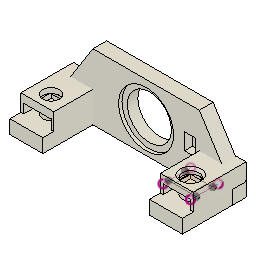
encoder-bracket (Autodesk Fusion 360 design; units mm, degrees)
Autodesk Fusion 360 part; units mm, degrees
sketch "Sketch1" plane through (0, 0, 0) normal (0, 0, 1) x (1, 0, 0)
  line L0 (-19.939, 0) -> (-19.939, 3.175)
  line L1 (-19.939, 3.175) -> (-12.319, 15.24)
  line L2 (-12.319, 15.24) -> (12.319, 15.24)
  line L3 (12.319, 15.24) -> (19.939, 3.175)
  line L4 (19.939, 3.175) -> (19.939, 0)
  line L5 (19.939, 0) -> (-19.939, 0)
  line L6 (0, 0) -> (0, 15.24) construction
  circle A0 centre (0, 7.3025) radius 5.08
  circle A1 centre (0, 7.3025) radius 6.35
  line L7 (8.89, 9.2075) -> (11.43, 9.2075)
  line L8 (11.43, 9.2075) -> (11.43, 5.3975)
  line L9 (11.43, 5.3975) -> (8.89, 5.3975)
  line L10 (8.89, 5.3975) -> (8.89, 9.2075)
  line L11 (10.16, 9.2075) -> (10.16, 5.3975) construction
  line L12 (0, 7.3025) -> (10.16, 7.3025) construction
  dimension "d1" = 39.878
  dimension "d2" = 3.175
  dimension "d3" = 7.62
  dimension "d4" = 15.24
  dimension "d5" = 10.16
  dimension "d6" = 7.3025
  dimension "d7" = 12.7
  dimension "d8" = 3.81
  dimension "d9" = 2.54
  dimension "d10" = 10.16
  constraint vertical L0
  constraint perpendicular L0 L2
  constraint perpendicular L2 L4
  constraint perpendicular L0 L5
  constraint midpoint L6.start L5
  constraint equal L0 L4
  constraint coincident L6.start origin
  constraint coincident L2 L6.end
  constraint perpendicular L2 L6
  constraint midpoint L2 L6.end
  constraint coincident L6 A0.centre
  constraint concentric A0 A1
  constraint horizontal L7
  constraint vertical L8
  constraint horizontal L9
  constraint vertical L10
  constraint midpoint L7 L11.start
  constraint midpoint L9 L11.end
  constraint coincident A0.centre A1.centre
  constraint coincident L11 L12.end
  constraint perpendicular L11 L12
  constraint midpoint L11 L12.end
  measures "d1" distance of L0.start L4.end
  measures "d2" distance of L0.start L0.end
  measures "d3" horizontal distance of L0.start L1.end
  measures "d4" distance of L2 L5
  measures "d5" diameter of A0
  measures "d6" distance of L6.start A0.centre
  measures "d7" diameter of A1
  measures "d8" distance of L7.end L8.end
  measures "d9" distance of L7.start L7.end
  measures "d10" distance of A0.centre L12.end
extrude "Extrude1" add sketch "Sketch1" against normal blind 3.175 contours L0 L1 L2 L3 L4 L5 | A1 | L7 L8 L9 L10 makes body 1
extrude "Extrude2" cut sketch "Sketch1" against normal blind 0.762 contours A1 bodies 1
extrude "Extrude3" cut sketch "Sketch1" against normal blind 1.905 contours L7 L8 L9 L10 bodies 1
sketch "Sketch3" plane through (0, 0, 0) normal (0, 1, 0) x (1, 0, 0)
  line L0 (19.939, 3.175) -> (12.319, 3.175)
  line L1 (12.319, 3.175) -> (12.319, -9.017)
  line L2 (12.319, -9.017) -> (19.939, -9.017)
  line L3 (19.939, -9.017) -> (19.939, 3.175)
  line L4 (12.319, -5.842) -> (19.939, -5.842) construction
  circle A0 centre (16.129, -5.842) radius 1.905
  line L5 (12.319, 0) -> (19.939, 0)
  line L6 (12.319, -9.017) -> (19.939, -9.017)
  line L7 (19.939, -9.017) -> (19.939, -11.557)
  line L8 (19.939, -11.557) -> (12.319, -11.557)
  line L9 (12.319, -11.557) -> (12.319, -9.017)
  point P0 (19.939, 3.175)
  dimension "d17" = 12.192
  dimension "d18" = 7.62
  dimension "d19" = 3.81
  dimension "d21" = 5.842
  dimension "d31" = 2.54
  constraint horizontal L0
  constraint vertical L1
  constraint horizontal L2
  constraint vertical L3
  constraint coincident L1 L4.start
  constraint coincident L3 L4.end
  constraint perpendicular L3 L4
  constraint midpoint L4 A0.centre
  constraint coincident P0 L0.start
  constraint horizontal L6
  constraint vertical L7
  constraint horizontal L8
  constraint vertical L9
  constraint equal L2 L8
  measures "d17" distance of P0 L2.end
  measures "d18" distance of L1.end L2.end
  measures "d19" diameter of A0
  measures "d21" distance of L4 L5
  measures "d31" distance of L2.end L7.end
extrude "Extrude4" add sketch "Sketch3" along normal blind 7.112 separate body contours L0 L1 L3 L5 | L1 L2 L3 L5 L6 makes body 2
extrude "Extrude6" add sketch "Sketch3" along normal blind 3.175 contours L2 L6 L7 L8 L9 bodies 2
sketch "Sketch4" plane through (0, 0, 9.017) normal (0, 0, 1) x (1, 0, 0)
  line L0 (19.939, 3.175) -> (19.939, 7.112)
  line L1 (19.939, 7.112) -> (12.319, 7.112)
  line L2 (12.319, 7.112) -> (12.319, 3.175)
  line L3 (12.954, 5.334) -> (19.304, 5.334)
  line L4 (19.304, 5.334) -> (19.304, 3.175)
  line L5 (12.954, 3.175) -> (12.954, 5.334)
  line L6 (16.129, 7.112) -> (16.129, 5.334) construction
  line L7 (12.319, 3.175) -> (19.939, 3.175)
  dimension "d24" = 6.35
  dimension "d25" = 2.159
  constraint horizontal L3
  constraint vertical L4
  constraint vertical L5
  constraint midpoint L1 L6.start
  constraint coincident L3 L6.end
  constraint perpendicular L3 L6
  constraint midpoint L3 L6.end
  constraint coincident L4.end L7
  constraint coincident L5.start L7
  measures "d24" distance of L3.start L3.end
  measures "d25" distance of L3.end L4.end
extrude "Extrude5" cut sketch "Sketch4" against normal blind 6.35 contours L3 L4 L5 L7 bodies 2
sketch "Sketch5" plane through (0, 5.334, 0) normal (0, -1, 0) x (1, 0, 0)
  circle A0 centre (16.129, 5.842) radius 1.905
  line L0 (19.304, 9.017) -> (12.954, 9.017)
  line L1 (12.954, 9.017) -> (12.954, 2.667)
  line L2 (12.954, 2.667) -> (19.304, 2.667)
  line L3 (19.304, 2.667) -> (19.304, 9.017)
  line L4 (12.954, 7.747) -> (19.304, 7.747)
  line L5 (19.304, 3.937) -> (12.954, 3.937)
  line L6 (12.954, 9.017) -> (12.954, 2.667)
  line L7 (19.304, 9.017) -> (19.304, 2.667)
  line L8 (18.034, 7.747) -> (18.034, 3.937)
  line L9 (14.224, 7.747) -> (14.224, 3.937)
  constraint horizontal L4
  constraint horizontal L5
  constraint tangent A0 L4
  constraint tangent A0 L5
  constraint coincident L1 L4.start
  constraint coincident L1 L5.end
  constraint coincident L3 L5.start
  constraint coincident L3 L4.end
  constraint vertical L8
  constraint tangent A0 L8
  constraint perpendicular L4 L9
  constraint tangent A0 L9
  constraint coincident L4 L9.start
  constraint coincident L4 L8.start
  constraint coincident L5 L8.end
  constraint coincident L5 L9.end
extrude "Extrude7" cut sketch "Sketch5" against normal blind 0.1999 contours A0 L5 L8 | A0 L4 L8 | L3 L4 L5 L7 L8 | A0 L4 L9 | A0 L5 L9 | L1 L4 L5 L6 L9 bodies 2
extrude "Extrude8" cut sketch "Sketch5" against normal blind 0.6 contours A0 L5 L8 | A0 L4 L8 | A0 L4 L9 | A0 L5 L9 bodies 2
chamfer "Chamfer1" distance 0.508 angle 45 2 edges at (14.3529, 7.112, 5.1531) (14.3529, 0, 5.1531) on bodies 2
mirror "Mirror1" about plane through (0, 0, 0) normal (1, 0, 0) of "Extrude4", "Extrude6", "Extrude5", "Extrude7", "Extrude8" makes body 3
